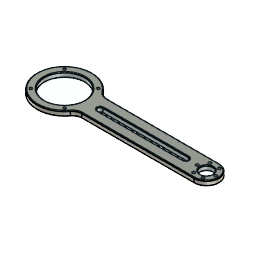
Upper Arm v4 (Autodesk Fusion 360 design; units mm, degrees)
Autodesk Fusion 360 part; units mm, degrees
note: some values were not read from the file. Set by a fixed rule: which sketch regions a step uses.
sketch "Sketch1" plane through (0, 0, 0) normal (0, 0, 1) x (1, 0, 0)
  circle A0 centre (0, 0) radius 32.1
  circle A1 centre (0, 0) radius 44
  line L0 (26.9905, -26.9905) -> (-26.9905, -26.9905)
  line L1 (-26.9905, -26.9905) -> (-26.9905, 26.9905)
  line L2 (-26.9905, 26.9905) -> (26.9905, 26.9905)
  line L3 (26.9905, 26.9905) -> (26.9905, -26.9905)
  line L4 (26.9905, -26.9905) -> (-26.9905, 26.9905) construction
  line L5 (-26.9905, -26.9905) -> (26.9905, 26.9905) construction
  circle A2 centre (-26.9905, -26.9905) radius 2
  line L6 (5, 0) -> (0, 0) construction
  line L7 (0, 0) -> (0, 5) construction
  circle A3 centre (-26.9905, 26.9905) radius 2
  circle A4 centre (26.9905, 26.9905) radius 2
  circle A5 centre (26.9905, -26.9905) radius 2
  line L8 (26.9905, 21.1832) -> (26.9905, -21.1832)
  line L9 (26.9905, 0) -> (26.9905, 20)
  line L10 (26.9905, 0) -> (26.9905, -20)
  line L11 (26.9905, 20) -> (226.9905, 20)
  line L12 (26.9905, -20) -> (226.9905, -20)
  circle A6 centre (226.9905, 0) radius 20
  circle A7 centre (226.9905, 0) radius 15
  line L13 (226.9905, 0) -> (241.9905, 0)
  circle A8 centre (241.9905, 0) radius 2.15
  circle A9 centre (234.4905, 12.9904) radius 2.15
  circle A10 centre (219.4905, 12.9904) radius 2.15
  circle A11 centre (211.9905, 0) radius 2.15
  circle A12 centre (219.4905, -12.9904) radius 2.15
  circle A13 centre (234.4905, -12.9904) radius 2.15
  line L14 (44, 0) -> (57, 0)
  line L15 (206.9905, 0.0088) -> (193.9905, 0.0088)
  circle A14 centre (57, 0) radius 4.3
  circle A15 centre (193.9905, 0.0088) radius 4.3
  line L16 (57, 0) -> (57, 4.3)
  line L17 (57, 4.3) -> (193.9902, 4.3088)
  line L18 (193.9905, -4.2912) -> (57.0003, -4.3)
  circle A16 centre (226.9905, 0) radius 10
  dimension "d1" = 64.2
  dimension "d2" = 88
  dimension "d3" = 53.981
  dimension "d4" = 53.981
  dimension "d5" = 4
  dimension "d6" = 5
  dimension "d7" = 5
  dimension "d84" = 20
  dimension "d86" = 20
  dimension "d88" = 200
  dimension "d89" = 200
  dimension "d90" = 30
  dimension "d91" = 4.3
  dimension "d93" = 360
  dimension "d94" = 13
  dimension "d95" = 13
  dimension "d96" = 8.6
  dimension "d97" = 8.6
  dimension "d98" = 20
  constraint coincident A0.centre A1.centre
  constraint concentric A0 A1
  constraint horizontal L0
  constraint perpendicular L0 L1
  constraint parallel L0 L2
  constraint parallel L1 L3
  constraint coincident L4 A0.centre
  constraint coincident L5 A0.centre
  constraint coincident L0.end L1.start
  constraint perpendicular L6 L7
  constraint symmetric A2 L6 A3
  constraint symmetric A2 L7 A5
  constraint symmetric L7 A3 A4
  constraint parallel L3 L8
  constraint midpoint L8 L9.start
  constraint parallel L3 L9
  constraint parallel L8 L10
  constraint perpendicular L8 L11
  constraint perpendicular L10 L12
  constraint coincident L12.end A6
  constraint tangent L12 A6
  constraint coincident L11.end A6
  constraint concentric A6 A7
  constraint coincident A6.centre A7.centre
  constraint coincident A7 L13.end
  constraint horizontal L13
  constraint coincident L13.end A8.centre
  constraint coincident A1 L14.start
  constraint horizontal L14
  constraint coincident A6 L15.start
  constraint parallel L11 L15
  constraint coincident L14.end A14.centre
  constraint coincident L15.end A15.centre
  constraint coincident A14 L16.end
  constraint perpendicular L14 L16
  constraint coincident A15 L17.end
  constraint tangent A15 L17
  constraint coincident A15 L18.start
  constraint coincident A14 L18.end
  constraint tangent A14 L18
  constraint concentric A6 A16
  measures "d1" diameter of A0
  measures "d2" diameter of A1
  measures "d3" distance of L1.end L2.end
  measures "d4" distance of L0.end L1.end
  measures "d5" diameter of A2
  measures "d6" distance of A0.centre L6.start
  measures "d7" distance of A0.centre L7.end
  measures "d84" distance of L9.start L9.end
  measures "d86" distance of L9.start L10.end
  measures "d88" distance of L9.end L11.end
  measures "d89" distance of L10.end L12.end
  measures "d90" diameter of A7
  measures "d91" diameter of A8
  measures "d94" distance of L14.start L14.end
  measures "d95" distance of L15.start L15.end
  measures "d96" diameter of A14
  measures "d97" diameter of A15
  measures "d98" diameter of A16
extrude "Extrude1" add sketch "Sketch1" along normal blind 8 contours A0 A1 L3 L8 L9 L10 L11 L12 | A0 L2 L3 A4 L8 L9 | A0 L0 L3 A5 L8 L10 | A0 A1 L0 L1 L2 L3 A2 A3 A4 A5 L8 L11 L12 | A0 L1 L2 A3 | A1 L11 A6 L14 L15 A14 A15 L17 | A0 L0 L1 A2 | A1 L12 A6 L14 L15 A14 A15 L18 | A6 | A7 A8 A9 A10 A11 A12 A13
fillet "Fillet25" radius 15 2 edges at (39.1918, -20, 4) (39.1918, 20, 4)
fillet "Fillet23" radius 1 20 edges at (133.0912, -20, 8) (246.9905, 0, 8) (133.0912, 20, 8) (-44, 0, 8) (-29.9277, 11.6079, 0) (-29.9277, 11.6079, 8) (133.0912, -20, 0) (246.9905, 0, 0) (133.0912, 20, 0) (-44, 0, 0) (217.6672, 3.6162, 8) (217.6672, 3.6162, 0) (125.4951, 4.3044, 0) (198.2905, 0.0089, 0) (125.4954, -4.2956, 0) (52.7, -0.0001, 0) (125.4951, 4.3044, 8) (198.2905, 0.0089, 8) (125.4954, -4.2956, 8) (52.7, -0.0001, 8)
sketch "Sketch6" plane through (0, 0, 8) normal (0, 0, 1) x (-1, 0, 0)
  circle A0 centre (-226.9905, 0) radius 11
  line L0 (-47.4974, 19) -> (-226.9905, 19)
  arc A1 (-226.9905, 19) -> (-226.9905, -19) centre (-226.9905, 0) ccw
  line L1 (-226.9905, -19) -> (-47.4974, -19)
  arc A2 (-34.6167, -25.5085) -> (-47.4974, -19) centre (-47.4974, -35) ccw
  arc A3 (-34.6167, -25.5085) -> (-34.6167, 25.5085) centre (0, 0) ccw
  arc A4 (-47.4974, 19) -> (-34.6167, 25.5085) centre (-47.4974, 35) ccw
  circle A5 centre (-219.4905, -12.9904) radius 2.15
  circle A6 centre (-234.4905, -12.9904) radius 2.15
  circle A7 centre (-219.4905, 12.9904) radius 2.15
  circle A8 centre (-234.4905, 12.9904) radius 2.15
  circle A9 centre (-241.9905, 0) radius 2.15
  circle A10 centre (26.9905, -26.9905) radius 2
  circle A11 centre (-211.9905, 0) radius 2.15
  circle A12 centre (26.9905, 26.9905) radius 2
  circle A13 centre (-26.9905, 26.9905) radius 2
  circle A14 centre (-26.9905, -26.9905) radius 2
  circle A15 centre (0, 0) radius 33.1
  line L2 (-56.9999, -5.3) -> (-193.9902, -5.3088)
  arc A16 (-193.9905, 5.2912) -> (-193.9902, -5.3088) centre (-193.9905, -0.0088) ccw
  line L3 (-193.9905, 5.2912) -> (-57.0003, 5.3)
  arc A17 (-57, -5.3) -> (-57.0003, 5.3) centre (-57, 0) ccw
